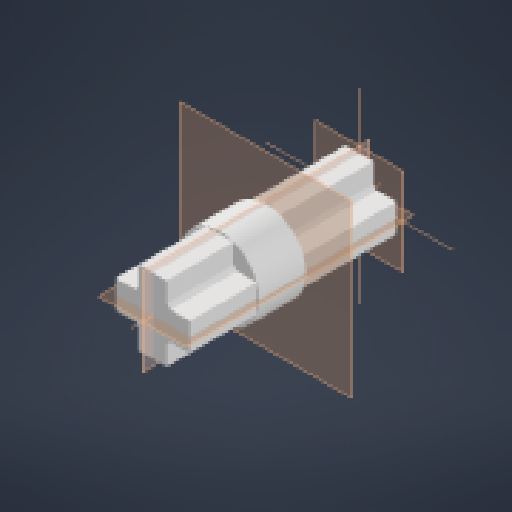
# Autodesk Inventor part: EjeCortoGrua
Saved by Autodesk Inventor 2026.2 (Build 302298010, 298A)
## iProperties
Created: 2026-04-22
Part Number: EjeCortoGrua
Material: Genérico
Document SubType Name: Modeling
Designer: Jose Carlos
Density: 1 g/cm^3
Appearance: Valor por defecto
Author: Jose Carlos
Autodesk Inventor part; units mm, degrees
sketch "Boceto1" plane through (0, 0, 0) normal (0, 0, 1) x (1, 0, 0)
  line L0 (-0.9, -2.4) -> (0.9, -2.4)
  line L1 (0.9, -2.4) -> (0.9, 2.4)
  line L2 (0.9, 2.4) -> (-0.9, 2.4)
  line L3 (-0.9, 2.4) -> (-0.9, -2.4)
  line L4 (-0.9, -2.4) -> (0.9, 2.4) construction
  line L5 (0.9, -2.4) -> (-0.9, 2.4) construction
  line L6 (2.4, -0.9) -> (-2.4, -0.9)
  line L7 (-2.4, -0.9) -> (-2.4, 0.9)
  line L8 (-2.4, 0.9) -> (2.4, 0.9)
  line L9 (2.4, 0.9) -> (2.4, -0.9)
  line L10 (2.4, -0.9) -> (-2.4, 0.9) construction
  line L11 (-2.4, -0.9) -> (2.4, 0.9) construction
  circle A0 centre (0, 0) radius 1.45
  point P0 (1.1369, 0.9)
  point P1 (0.9, 1.1369)
  point P2 (-0.9, 1.1369)
  point P3 (-1.1369, 0.9)
  point P4 (-1.1369, -0.9)
  point P5 (-0.9, -1.1369)
  point P6 (0.9, -1.1369)
  point P7 (1.1369, -0.9)
  dimension "d14" = 2.9
  dimension "d15" = 1.8
  dimension "d16" = 4.8
  constraints: 24 end point, 5 midpoint, 4 parallel, 4 perpendicular, 2 coincident, 2 horizontal, 1 centre point
  measures "d14" diameter of A0
  measures "d15" distance of L1.end L2.end
  measures "d16" distance of L0.end L1.end
extrude "Extrusión1" add sketch "Boceto1" along normal blind 13.31
ref_plane "Plano de trabajo1" through (0, 0, 6) normal (0, 0, 1) x (1, 0, 0)
sketch "Boceto2" plane through (0, 0, 6) normal (0, 0, 1) x (1, 0, 0)
  line L0 (2.4, 0.9) -> (1.1369, 0.9) construction
  circle A0 centre (0, 0) radius 2.5632
  constraints: 1 coincident, 3 other
extrude "Extrusión2" add sketch "Boceto2" along normal blind 3
